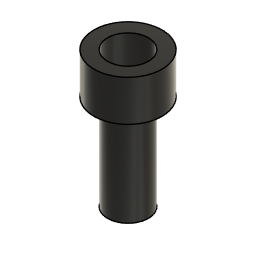
TORNILLOM3 (Autodesk Fusion 360 design; units mm, degrees)
Autodesk Fusion 360 part; units mm, degrees
sketch "Boceto1" plane through (0, 0, 0) normal (0, 0, 1) x (1, 0, 0)
  circle A0 centre (0, 0) radius 1.5
  dimension "d1" = 3
  constraint coincident A0.centre origin
  measures "d1" diameter of A0
extrude "Extruir1" add sketch "Boceto1" along normal blind 7 makes body 1
sketch "Boceto2" plane through (0, 0, 7) normal (0, 0, 1) x (-1, 0, 0)
  circle A0 centre (0, 0) radius 1.5
  circle A1 centre (0, 0) radius 2.5
  dimension "d4" = 5
  constraint concentric A0 A1
  measures "d4" diameter of A1
extrude "Extruir2" add sketch "Boceto2" along normal blind 3 separate body makes body 2
